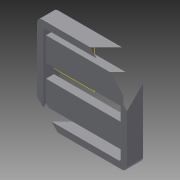
# Autodesk Inventor part: Case
Saved by Autodesk Inventor 2014 SP1 (Build 180222100, 222)
## iProperties
Created: 2014-04-19
Part Number: Case
Material: Aluminum 6061
Document SubType Name: Modeling
Designer: Ben
Density: 2.71 g/cm^3
Appearance: Aluminum - Flat
Author: Ben
Autodesk Inventor part; units mm, degrees
ref_plane "YZ Plane" through (0, 0, 0) normal (1, 0, 0) x (0, 1, 0)
ref_plane "XZ Plane" through (0, 0, 0) normal (0, 1, 0) x (-1, 0, 0)
ref_plane "XY Plane" through (0, 0, 0) normal (0, 0, 1) x (1, 0, 0)
ref_plane "Work Plane1" through (0, 0, 0) normal (0, 0, 1) x (1, 0, 0)
sketch "Sketch1" plane through (0, 0, 0) normal (0, 0, 1) x (1, 0, 0)
  line L0 (35.585, -35.585) -> (35.585, 35.585) projected
  line L1 (-35.585, -35.585) -> (35.585, -35.585) projected
  line L2 (35.615, -35.585) -> (106.785, -35.585) projected
  line L3 (35.615, -35.615) -> (35.615, -106.785) projected
  line L4 (-35.585, 35.585) -> (-35.585, -35.585) projected
  line L5 (35.585, 35.585) -> (-35.585, 35.585) projected
  line L6 (106.785, 35.585) -> (35.615, 35.585) projected
  line L7 (106.785, -35.585) -> (106.785, 35.585) projected
  line L8 (35.585, -35.585) -> (35.615, -35.615)
  line L9 (35.615, -35.585) -> (35.585, -35.615)
  line L10 (35.585, 35.8807) -> (107.085, 35.8807) construction
  line L11 (-35.915, 35.8807) -> (-35.915, 36.8807)
  line L12 (104.585, 37.3807) -> (-33.415, 37.3807)
  line L13 (-37.415, 33.3807) -> (-37.415, -104.6193)
  line L14 (-33.415, -108.6193) -> (104.585, -108.6193)
  line L15 (108.585, -104.6193) -> (108.585, 33.3807)
  arc A0 (104.585, -108.6193) -> (108.585, -104.6193) centre (104.585, -104.6193) ccw
  arc A1 (-37.415, -104.6193) -> (-33.415, -108.6193) centre (-33.415, -104.6193) ccw
  arc A2 (-33.415, 37.3807) -> (-37.415, 33.3807) centre (-33.415, 33.3807) ccw
  arc A3 (108.585, 33.3807) -> (104.585, 37.3807) centre (104.585, 33.3807) ccw
  line L16 (35.6, 49.4) -> (-39.4, 49.4)
  line L17 (120.6, 39.4) -> (120.6, -110.6)
  line L18 (110.6, -120.6) -> (-39.4, -120.6)
  line L19 (-49.4, -110.6) -> (-49.4, 39.4)
  arc A4 (-39.4, 49.4) -> (-49.4, 39.4) centre (-39.4, 39.4) ccw
  arc A5 (120.6, 39.4) -> (110.6, 49.4) centre (110.6, 39.4) ccw
  arc A6 (110.6, -120.6) -> (120.6, -110.6) centre (110.6, -110.6) ccw
  arc A7 (-49.4, -110.6) -> (-39.4, -120.6) centre (-39.4, -110.6) ccw
  line L20 (35.6, 49.4) -> (110.6, 49.4)
  point P0 (0, 0)
  point P1 (120.6, -120.6)
  point P2 (120.6, 49.4)
  point P3 (-49.4, -120.6)
  dimension "d2" = 71.5
  dimension "d15" = 1
  dimension "d18" = 4
  dimension "d21" = 170
  dimension "d22" = 170
  dimension "d23" = 10
  constraints: 26 end point, 16 point on circle, 16 tangent, 8 centre point, 6 equal radius, 6 point on line, 3 parallel, 3 perpendicular, 1 horizontal
  measures "d2" distance of L10.start L11.start
  measures "d15" distance of L11.start L11.end
  measures "d18" radius of A0
  measures "d21" distance of point (120.6, -120.6) point (-49.4, -120.6)
  measures "d22" distance of point (120.6, 49.4) point (120.6, -120.6)
  measures "d23" radius of A4
extrude "Extrusion2" add sketch "Sketch1" against normal blind 10 contours L20 A5 L17 A6 L18 A7 L19 A4 L16
sketch "Sketch3" plane through (0, 0, 0) normal (0, 0, 1) x (1, 0, 0)
  arc A0 (104.585, -108.6193) -> (108.585, -104.6193) centre (104.585, -104.6193) ccw projected
  line L0 (104.585, -108.6193) -> (-33.415, -108.6193) projected
  arc A1 (-37.415, -104.6193) -> (-33.415, -108.6193) centre (-33.415, -104.6193) ccw projected
  line L1 (-37.415, -104.6193) -> (-37.415, 33.3807) projected
  arc A2 (-33.415, 37.3807) -> (-37.415, 33.3807) centre (-33.415, 33.3807) ccw projected
  line L2 (-33.415, 37.3807) -> (104.585, 37.3807) projected
  arc A3 (108.585, 33.3807) -> (104.585, 37.3807) centre (104.585, 33.3807) ccw projected
  line L3 (108.585, 33.3807) -> (108.585, -104.6193) projected
  line L4 (110.6, 49.4) -> (-39.4, 49.4) projected
  arc A4 (-39.4, 49.4) -> (-49.4, 39.4) centre (-39.4, 39.4) ccw projected
  line L5 (-49.4, 39.4) -> (-49.4, -110.6) projected
  arc A5 (-49.4, -110.6) -> (-39.4, -120.6) centre (-39.4, -110.6) ccw projected
  line L6 (-39.4, -120.6) -> (110.6, -120.6) projected
  arc A6 (110.6, -120.6) -> (120.6, -110.6) centre (110.6, -110.6) ccw projected
  line L7 (120.6, -110.6) -> (120.6, 39.4) projected
  arc A7 (120.6, 39.4) -> (110.6, 49.4) centre (110.6, 39.4) ccw projected
  line L8 (108.585, -93.6) -> (-37.415, -93.6)
  line L9 (-37.415, -48.6) -> (108.585, -48.6)
  line L10 (108.585, 22.4) -> (-37.415, 22.4)
  line L11 (-37.415, -22.6) -> (108.585, -22.6)
  line L12 (108.585, 22.4) -> (108.585, -22.6)
  line L13 (-37.415, 22.4) -> (-37.415, -22.6)
  line L14 (-37.415, -48.6) -> (-37.415, -93.6)
  line L15 (108.585, -48.6) -> (108.585, -93.6)
  point P0 (0, 0)
  dimension "d27" = 45
  constraints: 16 end point, 4 point on line, 3 collinear, 2 perpendicular
  measures "d27" distance of L8.end L9.start
extrude "Extrusion3" add sketch "Sketch3" along normal blind 20 contours L8 L1 L9 L3 | L11 L1 L10 L3 | A7 L7 A6 L6 A5 L5 A4 L4
sketch "Sketch5" plane through (0, 0, -10) normal (0, 0, -1) x (-1, 0, 0)
  arc A0 (-108.585, -104.6193) -> (-104.585, -108.6193) centre (-104.585, -104.6193) ccw projected
  line L0 (-108.585, -104.6193) -> (-108.585, 33.3807) projected
  arc A1 (-104.585, 37.3807) -> (-108.585, 33.3807) centre (-104.585, 33.3807) ccw projected
  line L1 (-104.585, 37.3807) -> (33.415, 37.3807) projected
  arc A2 (37.415, 33.3807) -> (33.415, 37.3807) centre (33.415, 33.3807) ccw projected
  line L2 (37.415, 33.3807) -> (37.415, -104.6193) projected
  arc A3 (33.415, -108.6193) -> (37.415, -104.6193) centre (33.415, -104.6193) ccw projected
  line L3 (33.415, -108.6193) -> (-104.585, -108.6193) projected
  line L4 (33.415, 41.3807) -> (-104.585, 41.3807)
  arc A4 (-104.585, 41.3807) -> (-112.585, 33.3807) centre (-104.585, 33.3807) ccw
  line L5 (-112.585, 33.3807) -> (-112.585, -104.6193)
  arc A5 (-112.585, -104.6193) -> (-104.585, -112.6193) centre (-104.585, -104.6193) ccw
  line L6 (-104.585, -112.6193) -> (33.415, -112.6193)
  arc A6 (33.415, -112.6193) -> (41.415, -104.6193) centre (33.415, -104.6193) ccw
  line L7 (41.415, -104.6193) -> (41.415, 33.3807)
  arc A7 (41.415, 33.3807) -> (33.415, 41.3807) centre (33.415, 33.3807) ccw
  point P0 (0, 0)
  dimension "d32" = 4
  constraints: 8 end point, 8 point on circle, 4 centre point, 7 other
  measures "d32" distance between parallel lines of L1 L4
extrude "Extrusion5" cut sketch "Sketch5" against normal blind 3
sketch "Sketch6" plane through (0, 0, -10) normal (0, 0, -1) x (-1, 0, 0)
  line L0 (39.4, 49.4) -> (-110.6, 49.4) projected
  arc A0 (-110.6, 49.4) -> (-120.6, 39.4) centre (-110.6, 39.4) ccw projected
  line L1 (-120.6, 39.4) -> (-120.6, -110.6) projected
  arc A1 (-120.6, -110.6) -> (-110.6, -120.6) centre (-110.6, -110.6) ccw projected
  line L2 (-110.6, -120.6) -> (39.4, -120.6) projected
  arc A2 (39.4, -120.6) -> (49.4, -110.6) centre (39.4, -110.6) ccw projected
  line L3 (49.4, -110.6) -> (49.4, 39.4) projected
  arc A3 (49.4, 39.4) -> (39.4, 49.4) centre (39.4, 39.4) ccw projected
  line L4 (-110.6, 45.4) -> (39.4, 45.4)
  arc A4 (45.4, 39.4) -> (39.4, 45.4) centre (39.4, 39.4) ccw
  line L5 (45.4, 39.4) -> (45.4, -110.6)
  arc A5 (39.4, -116.6) -> (45.4, -110.6) centre (39.4, -110.6) ccw
  line L6 (39.4, -116.6) -> (-110.6, -116.6)
  arc A6 (-116.6, -110.6) -> (-110.6, -116.6) centre (-110.6, -110.6) ccw
  line L7 (-116.6, -110.6) -> (-116.6, 39.4)
  arc A7 (-110.6, 45.4) -> (-116.6, 39.4) centre (-110.6, 39.4) ccw
  point P0 (0, 0)
  dimension "d35" = 4
  constraints: 8 end point, 8 point on circle, 4 centre point, 7 other
  measures "d35" distance between parallel lines of L4 L0
extrude "Extrusion6" cut sketch "Sketch6" against normal blind 15
sketch "Sketch7" plane through (0, 0, 20) normal (0, 0, 1) x (1, 0, 0)
  line L0 (110.6, 49.4) -> (-39.4, 49.4) projected
  arc A0 (-39.4, 49.4) -> (-49.4, 39.4) centre (-39.4, 39.4) ccw projected
  line L1 (-49.4, 39.4) -> (-49.4, -110.6) projected
  arc A1 (-49.4, -110.6) -> (-39.4, -120.6) centre (-39.4, -110.6) ccw projected
  line L2 (-39.4, -120.6) -> (110.6, -120.6) projected
  arc A2 (110.6, -120.6) -> (120.6, -110.6) centre (110.6, -110.6) ccw projected
  line L3 (120.6, -110.6) -> (120.6, 39.4) projected
  arc A3 (120.6, 39.4) -> (110.6, 49.4) centre (110.6, 39.4) ccw projected
  line L4 (-39.4, 45.4) -> (110.6, 45.4)
  arc A4 (116.6, 39.4) -> (110.6, 45.4) centre (110.6, 39.4) ccw
  line L5 (116.6, 39.4) -> (116.6, -110.6)
  arc A5 (110.6, -116.6) -> (116.6, -110.6) centre (110.6, -110.6) ccw
  line L6 (110.6, -116.6) -> (-39.4, -116.6)
  arc A6 (-45.4, -110.6) -> (-39.4, -116.6) centre (-39.4, -110.6) ccw
  line L7 (-45.4, -110.6) -> (-45.4, 39.4)
  arc A7 (-39.4, 45.4) -> (-45.4, 39.4) centre (-39.4, 39.4) ccw
  point P0 (0, 0)
  dimension "d38" = 4
  constraints: 8 end point, 8 point on circle, 4 centre point, 7 other
  measures "d38" distance between parallel lines of L4 L0
extrude "Extrusion7" cut sketch "Sketch7" against normal blind 10
body "Solid2"
